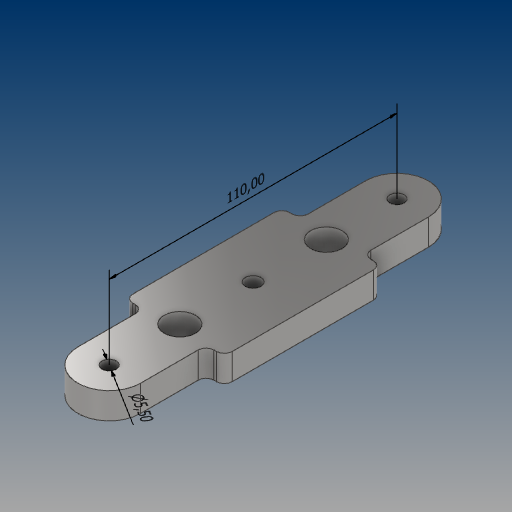
# Autodesk Inventor part: 04_Mieng_go_dem_lo_xo
Saved by Autodesk Inventor 2021 (Build 250183000, 183)
## iProperties
Created: 2024-04-04
Part Number: 04_Mieng_go_dem_lo_xo
Material: Stainless Steel, Austenitic
Document SubType Name: Modeling
Designer: Admin
Density: 8 g/cm^3
Appearance: Semi-Polished
Author: Admin
Autodesk Inventor part; units mm, degrees
ref_plane "YZ Plane" through (0, 0, 0) normal (1, 0, 0) x (0, 1, 0)
ref_plane "XZ Plane" through (0, 0, 0) normal (0, 1, 0) x (-1, 0, 0)
ref_plane "XY Plane" through (0, 0, 0) normal (0, 0, 1) x (1, 0, 0)
sketch "Sketch1" plane through (0, 0, 0) normal (0, 1, 0) x (-1, 0, 0)
  line L0 (0, 55) -> (0, -55) construction
  line L1 (-12, 55) -> (-12, -55)
  line L2 (12, -55) -> (12, 55)
  arc A0 (12, 55) -> (-12, 55) centre (0, 55) ccw
  arc A1 (-12, -55) -> (12, -55) centre (0, -55) ccw
  line L3 (-19, 30) -> (-19, -30)
  line L4 (-19, -30) -> (19, -30)
  line L5 (19, -30) -> (19, 30)
  line L6 (19, 30) -> (-19, 30)
  line L7 (-19, 30) -> (19, -30) construction
  line L8 (-19, -30) -> (19, 30) construction
  point P0 (0, 0)
  point P1 (-12, 30)
  point P2 (-12, -30)
  point P3 (12, -30)
  point P4 (12, 30)
  dimension "d0" = 60
  dimension "d1" = 110
  dimension "d2" = 12
  dimension "d3" = 38
  constraints: 20 end point, 4 point on circle, 4 tangent, 3 midpoint, 3 parallel, 2 centre point, 2 vertical, 1 perpendicular
  measures "d0" distance of L4.end L5.end
  measures "d1" distance of L0.start L0.end
  measures "d2" radius of A1
  measures "d3" distance of L3.end L4.end
extrude "Extrusion1" add sketch "Sketch1" along normal blind 10
sketch "Sketch2" plane through (0, 10, 0) normal (0, 1, 0) x (1, 0, 0)
  line L0 (19, -30) -> (19, 30) projected
  line L1 (19, 30) -> (12, 30) projected
  line L2 (12, 30) -> (12, 55) projected
  arc A0 (12, 55) -> (-12, 55) centre (0, 55) ccw projected
  line L3 (-12, 55) -> (-12, 30) projected
  line L4 (-12, 30) -> (-19, 30) projected
  line L5 (-19, 30) -> (-19, -30) projected
  line L6 (-19, -30) -> (-12, -30) projected
  line L7 (-12, -30) -> (-12, -55) projected
  arc A1 (-12, -55) -> (12, -55) centre (0, -55) ccw projected
  line L8 (12, -55) -> (12, -30) projected
  line L9 (12, -30) -> (19, -30) projected
  line L10 (0, -28) -> (0, 28)
  line L11 (0, 0) -> (-19, 0)
  line L12 (-19, 30) -> (-19, -30) projected
  dimension "d6" = 56
  constraints: 4 end point, 2 midpoint, 1 symmetric about line, 1 vertical
  measures "d6" distance of L10.start L10.end
hole "Hole1" at (0, 10, 28) at (0, 10, -28) direction (0, -1, 0) diameter 12 end through all
fillet "Fillet1" radius 3 8 edges at (19, 5, 30) (19, 5, -30) (12, 5, 30) (-19, 5, 30) (-12, 5, 30) (-19, 5, -30) (-12, 5, -30) (12, 5, -30)
sketch "Sketch3" plane through (0, 10, 0) normal (0, 1, 0) x (1, 0, 0)
  arc A0 (-12, -55) -> (12, -55) centre (0, -55) ccw projected
  arc A1 (12, 55) -> (-12, 55) centre (0, 55) ccw projected
  point P0 (0, 0)
hole "Hole2" at (0, 10, 55) at (0, 10, -55) direction (0, -1, 0) diameter 5.5 end through all
sketch "Sketch4" plane through (0, 10, 0) normal (0, 1, 0) x (1, 0, 0)
  circle A0 centre (0, 0) radius 3
  dimension "d22" = 6
  constraints: 1 centre point, 1 coincident
  measures "d22" diameter of A0
extrude "Extrusion2" cut sketch "Sketch4" against normal blind 7.5
body "Solid1"
